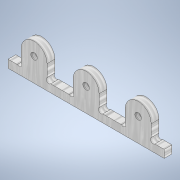
# Autodesk Inventor part: T字金具M3long
Saved by Autodesk Inventor 2020.2 (Build 242310000, 310)
## iProperties
Created: 2020-03-24
Part Number: T字金具M3long
Material: アルミニウム 7075
Document SubType Name: Modeling
Designer: aoyam
Density: 2.81 g/cm^3
Appearance: サテン - ブラシ仕上げ 重厚
Author: aoyam
Autodesk Inventor part; units mm, degrees
ref_plane "YZ Plane" through (0, 0, 0) normal (1, 0, 0) x (0, 1, 0)
ref_plane "XZ Plane" through (0, 0, 0) normal (0, 1, 0) x (-1, 0, 0)
ref_plane "XY Plane" through (0, 0, 0) normal (0, 0, 1) x (1, 0, 0)
sketch "スケッチ1" plane through (0, 0, 0) normal (0, 0, 1) x (1, 0, 0)
  circle A0 centre (0, 0) radius 1.25
  circle A1 centre (0, 0) radius 5
  line L0 (-10, -6) -> (10, -6)
  line L1 (10, -6) -> (10, -9)
  line L2 (10, -9) -> (-10, -9)
  line L3 (-10, -9) -> (-10, -6)
  line L4 (-5, 0) -> (-5, -6)
  line L5 (5, 0) -> (5, -6)
  circle A2 centre (-5.7106, -5.2894) radius 1.005
  circle A3 centre (5.7106, -5.2894) radius 1.005
  line L6 (-5.7106, -5.2894) -> (-5, -6)
  line L7 (5.7106, -5.2894) -> (5, -6)
  line L8 (-25, 0) -> (-25, -6)
  line L9 (-30, -6) -> (-10, -6)
  line L10 (-10, -9) -> (-30, -9)
  circle A4 centre (-20, 0) radius 5
  line L11 (-14.2894, -5.2894) -> (-15, -6)
  circle A5 centre (-14.2894, -5.2894) radius 1.005
  line L12 (-15, 0) -> (-15, -6)
  line L13 (-10, -6) -> (-10, -9)
  circle A6 centre (-20, 0) radius 1.25
  line L14 (-25.7106, -5.2894) -> (-25, -6)
  circle A7 centre (-25.7106, -5.2894) radius 1.005
  line L15 (-30, -9) -> (-30, -6)
  line L16 (-45, 0) -> (-45, -6)
  line L17 (-50, -6) -> (-30, -6)
  line L18 (-30, -9) -> (-50, -9)
  circle A8 centre (-40, 0) radius 5
  line L19 (-34.2894, -5.2894) -> (-35, -6)
  circle A9 centre (-34.2894, -5.2894) radius 1.005
  line L20 (-35, 0) -> (-35, -6)
  line L21 (-30, -6) -> (-30, -9)
  circle A10 centre (-40, 0) radius 1.25
  line L22 (-45.7106, -5.2894) -> (-45, -6)
  circle A11 centre (-45.7106, -5.2894) radius 1.005
  line L23 (-50, -9) -> (-50, -6)
  point P0 (6.4213, -6)
  point P1 (5, -4.5787)
  point P2 (-5, -4.5787)
  point P3 (-6.4213, -6)
  point P4 (-45, -4.5787)
  point P5 (-46.4213, -6)
  point P6 (6.4213, -6)
  point P7 (5, -4.5787)
  point P8 (-5, -4.5787)
  point P9 (-6.4213, -6)
  point P10 (-13.5787, -6)
  point P11 (-15, -4.5787)
  point P12 (-25, -4.5787)
  point P13 (-26.4213, -6)
  point P14 (-33.5787, -6)
  point P15 (-35, -4.5787)
  dimension "d7" = 2.01
  dimension "d8" = 2.01
  dimension "d0" = 2.5
  dimension "d1" = 10
  dimension "d2" = 3
  dimension "d3" = 20
  dimension "d4" = 6
  dimension "d5" = 5
  dimension "d6" = 6
  dimension "d9" = 45
  dimension "d10" = 45
  dimension "d13" = 20
  constraints: 48 end point, 9 coincident, 6 centre point, 6 horizontal, 6 point on circle, 6 point on line, 5 perpendicular, 1 collinear, 1 tangent, 65 other
  measures "d0" diameter of A0
  measures "d1" diameter of A1
  measures "d2" distance of L0.end L1.end
  measures "d3" distance of L1.end L2.end
  measures "d4" distance from line of L0 A1.centre
  measures "d5" distance of L0.end L5.end
  measures "d6" distance of L4.start L4.end
  measures "d9" angle of L4 L6
  measures "d10" angle of L5 L7
  measures "d13" distance of L4.start L8.start
extrude "押し出し1" add sketch "スケッチ1" along normal blind 3 contours A1 | L5 A3 L0 A2 L4 A1 | A3 L0 L1 L2 L3 A2 | L3 L10 L15 L9 A7 A5 | L18 L23 L17 A11 A9 L15 | L9 A7 L8 A4 L12 A5 | A4 | L17 A11 L16 A8 L20 A9 | A8
thread "ねじ1" size "M3x0.5" class "6H" standard "ANSI Metric M Profile" full length
thread "ねじ2" size "M3x0.5" class "6H" standard "ANSI Metric M Profile" full length
thread "ねじ3" size "M3x0.5" class "6H" standard "ANSI Metric M Profile" full length
